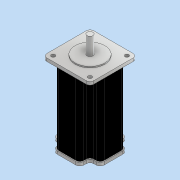
# Autodesk Inventor part: Silnik krokowy SM 60 100-4004AF - 4Nm
Saved by Autodesk Inventor 2018 (Build 220112000, 112)
## iProperties
Created: 2019-01-23
Part Number: Silnik krokowy SM 60 100-4004AF - 4Nm
Material: Ogólny
Document SubType Name: Modeling
Designer: Dawid
Density: 1 g/cm^3
Appearance: Aluminium — ciemne
Author: Dawid
Autodesk Inventor part; units mm, degrees
ref_plane "YZ Plane" through (0, 0, 0) normal (1, 0, 0) x (0, 1, 0)
ref_plane "XZ Plane" through (0, 0, 0) normal (0, 1, 0) x (-1, 0, 0)
ref_plane "XY Plane" through (0, 0, 0) normal (0, 0, 1) x (1, 0, 0)
sketch "Szkic1" plane through (0, 0, 0) normal (0, 0, 1) x (1, 0, 0)
  line L0 (-30, -30) -> (30, -30)
  line L1 (30, -30) -> (30, 30)
  line L2 (30, 30) -> (-30, 30)
  line L3 (-30, 30) -> (-30, -30)
  line L4 (-30, -30) -> (30, 30) construction
  line L5 (30, -30) -> (-30, 30) construction
  point P0 (0, 0)
  dimension "d0" = 60
  dimension "d1" = 60
  constraints: 12 end point, 2 midpoint, 2 parallel, 1 horizontal, 1 perpendicular
  measures "d0" distance of L2.end L1.end
  measures "d1" distance of L1.end L0.end
extrude "Wyciągnięcie proste1" add sketch "Szkic1" along normal blind 100
sketch "Szkic2" plane through (0, 0, 100) normal (0, 0, 1) x (1, 0, 0)
  circle A0 centre (0, 0) radius 19.05
  dimension "d4" = 38.1
  constraints: 1 centre point, 1 coincident
  measures "d4" diameter of A0
extrude "Wyciągnięcie proste2" add sketch "Szkic2" along normal blind 1.6
sketch "Szkic3" plane through (0, 0, 100) normal (0, 0, 1) x (1, 0, 0)
  line L0 (0, 0) -> (0, 23.57)
  line L1 (30, -30) -> (30, 30) projected
  line L2 (-30, 30) -> (-30, -30) projected
  line L3 (0, 0) -> (0, -23.57)
  line L4 (0, -23.57) -> (23.57, -23.57)
  line L5 (0, -23.57) -> (-23.57, -23.57)
  line L6 (0, 23.57) -> (-23.57, 23.57)
  line L7 (0, 23.57) -> (23.57, 23.57)
  circle A0 centre (23.57, 23.57) radius 2.5
  circle A1 centre (-23.57, 23.57) radius 2.5
  circle A2 centre (-23.57, -23.57) radius 2.5
  circle A3 centre (23.57, -23.57) radius 2.5
  dimension "d13" = 47.14
  dimension "d14" = 47.14
  dimension "d15" = 47.14
  dimension "d16" = 5
  dimension "d17" = 5
  dimension "d18" = 5
  dimension "d19" = 5
  constraints: 12 end point, 4 centre point, 4 coincident, 4 horizontal, 1 point on line, 1 vertical
  measures "d13" distance of L7.end L6.end
  measures "d14" distance of L4.end L5.end
  measures "d15" distance of L4.end L7.end
  measures "d16" diameter of A0
  measures "d17" diameter of A1
  measures "d18" diameter of A2
  measures "d19" diameter of A3
extrude "Wyciągnięcie proste3" cut sketch "Szkic3" against normal up to next
sketch "Szkic4" plane through (0, 0, 0) normal (0, 0, -1) x (-1, 0, 0)
  circle A0 centre (23.57, -23.57) radius 2.5 projected
  circle A1 centre (-23.57, 23.57) radius 2.5 projected
  circle A2 centre (23.57, 23.57) radius 2.5 projected
  circle A3 centre (-23.57, -23.57) radius 2.5 projected
  line L0 (30, -30) -> (-30, -30) projected
  line L1 (30, 30) -> (30, -30) projected
  line L2 (-30, 30) -> (30, 30) projected
  line L3 (-30, -30) -> (-30, 30) projected
  line L4 (-30, -30) -> (-30, 30) projected
  line L5 (-17, -17) -> (-17, -30)
  line L6 (17, -17) -> (17, -30)
  line L7 (30, 30) -> (30, -30) projected
  line L8 (-17, -17) -> (-30, -17)
  line L9 (17, 17) -> (30, 17)
  line L10 (-17, 17) -> (-17, 30)
  line L11 (-17, 17) -> (-30, 17)
  line L12 (17, 17) -> (17, 30)
  line L13 (17, -17) -> (30, -17)
  point P0 (0, 0)
  constraints: 16 end point, 8 point on line, 2 parallel, 2 perpendicular
extrude "Wyciągnięcie proste4" cut sketch "Szkic4" against normal blind 96 contours L0 L6 L13 L1 | L0 L3 L8 L5 | L9 L12 L2 L1 | L3 L2 L10 L11
sketch "Szkic5" plane through (0, 0, 101.6) normal (0, 0, 1) x (1, 0, 0)
  circle A0 centre (0, 0) radius 3.75
  dimension "d25" = 7.5
  constraints: 1 centre point, 1 coincident
  measures "d25" diameter of A0
extrude "Wyciągnięcie proste5" add sketch "Szkic5" along normal blind 22.5
sketch "Szkic6" plane through (-30, 30, 100) normal (0, 1, 0) x (1, 0, 0)
  line L0 (13, 100) -> (13, 4) projected
  line L1 (13, 4) -> (0, 4) projected
  line L2 (0, 4) -> (0, 0) projected
  line L3 (60, 0) -> (0, 0) projected
  line L4 (60, 4) -> (60, 0) projected
  line L5 (60, 4) -> (47, 4) projected
  line L6 (47, 4) -> (47, 100) projected
  line L7 (47, 100) -> (13, 100) projected
  line L8 (13, 4) -> (47, 4)
  line L9 (13, 100) -> (13, 4) projected
  line L10 (13, 100) -> (13, 96)
  line L11 (13, 96) -> (47, 96)
  point P0 (30, 100)
  dimension "d28" = 4
  constraints: 6 end point, 2 point on line, 1 horizontal, 1 perpendicular
  measures "d28" distance of L0.start L10.end
extrude "Wyciągnięcie proste6" cut sketch "Szkic6" against normal blind 1 contours L11 L6 L8 L0
sketch "Szkic7" plane through (-30, -30, 100) normal (-1, 0, 0) x (0, 0, 1)
  line L0 (-4, 47) -> (-100, 47) projected
  line L1 (-100, 47) -> (-100, 13) projected
  line L2 (-100, 13) -> (-4, 13) projected
  line L3 (-4, 13) -> (-4, 0) projected
  line L4 (-4, 0) -> (0, 0) projected
  line L5 (0, 60) -> (0, 0) projected
  line L6 (-4, 60) -> (0, 60) projected
  line L7 (-4, 60) -> (-4, 47) projected
  line L8 (-100, 47) -> (-4, 47) projected
  line L9 (-100, 13) -> (-4, 13) projected
  line L10 (-4, 47) -> (-4, 13)
  line L11 (-100, 47) -> (-100, 13) projected
  line L12 (-96, 13) -> (-96, 47)
  point P0 (-100, 30)
  constraints: 4 end point, 2 point on line, 1 perpendicular, 1 vertical
sketch "Szkic8" plane through (-30, -30, 100) normal (0, -1, 0) x (1, 0, 0)
  line L0 (13, -4) -> (13, -100) projected
  line L1 (13, -100) -> (47, -100) projected
  line L2 (47, -100) -> (47, -4) projected
  line L3 (47, -4) -> (60, -4) projected
  line L4 (60, -4) -> (60, 0) projected
  line L5 (0, 0) -> (60, 0) projected
  line L6 (0, -4) -> (0, 0) projected
  line L7 (0, -4) -> (13, -4) projected
  line L8 (47, -4) -> (13, -4) projected
  line L9 (13, -4) -> (47, -4)
  line L10 (47, -100) -> (47, -96)
  line L11 (47, -100) -> (47, -4) projected
  line L12 (47, -96) -> (13, -96)
  point P0 (30, -100)
  dimension "d34" = 4
  constraints: 6 end point, 2 point on line, 1 horizontal, 1 perpendicular
  measures "d34" distance of L1.end L10.end
sketch "Szkic9" plane through (30, -30, 100) normal (1, 0, 0) x (0, 0, -1)
  line L0 (4, 13) -> (100, 13) projected
  line L1 (100, 13) -> (100, 47) projected
  line L2 (100, 47) -> (4, 47) projected
  line L3 (4, 47) -> (4, 60) projected
  line L4 (4, 60) -> (0, 60) projected
  line L5 (0, 0) -> (0, 60) projected
  line L6 (4, 0) -> (0, 0) projected
  line L7 (4, 0) -> (4, 13) projected
  line L8 (4, 47) -> (4, 13) projected
  line L9 (4, 13) -> (4, 47)
  line L10 (100, 47) -> (100, 60) projected
  line L11 (100, 47) -> (96, 47)
  line L12 (100, 47) -> (4, 47) projected
  line L13 (96, 47) -> (96, 13)
  line L14 (100, 13) -> (4, 13) projected
  point P0 (100, 30)
  dimension "d37" = 4
  constraints: 6 end point, 2 point on line, 1 perpendicular, 1 vertical
  measures "d37" distance of L1.end L11.end
extrude "Wyciągnięcie proste10" cut sketch "Szkic8" against normal blind 1 contours L8 L2 L12 L0
extrude "Wyciągnięcie proste11" cut sketch "Szkic7" against normal blind 1 contours L10 L2 L12 L0
extrude "Wyciągnięcie proste12" cut sketch "Szkic9" against normal blind 1 contours L8 L2 L13 L0
sketch "Szkic10" plane through (-30, 17, 0) normal (0, 1, 0) x (1, 0, 0)
  line L0 (1, -4) -> (1, -96)
  line L1 (1, -96) -> (13, -96)
  line L2 (13, -4) -> (13, -96)
  line L3 (1, -4) -> (1, -96)
  line L4 (1, -4) -> (13, -4)
  point P0 (30, 0)
  constraints: 10 end point
extrude "Wyciągnięcie proste13" cut sketch "Szkic10" against normal blind 1
sketch "Szkic11" plane through (-17, 17, 0) normal (-1, 0, 0) x (0, 0, 1)
  line L0 (4, 0) -> (4, -1)
  line L1 (4, -1) -> (96, -1)
  line L2 (96, -1) -> (96, 12)
  line L3 (96, 12) -> (4, 12)
  line L4 (96, 12) -> (4, 12)
  line L5 (4, 12) -> (4, 0)
  point P0 (0, -17)
  constraints: 12 end point
extrude "Wyciągnięcie proste14" cut sketch "Szkic11" against normal blind 1
sketch "Szkic12" plane through (17, 17, 0) normal (0, 1, 0) x (1, 0, 0)
  line L0 (12, -96) -> (12, -4)
  line L1 (0, -4) -> (0, -96)
  line L2 (0, -96) -> (12, -96)
  line L3 (12, -4) -> (0, -4)
  point P0 (-17, 0)
  constraints: 8 end point
extrude "Wyciągnięcie proste15" cut sketch "Szkic12" against normal blind 1
sketch "Szkic13" plane through (17, 17, 0) normal (1, 0, 0) x (0, 0, -1)
  line L0 (-4, 12) -> (-96, 12)
  line L1 (-96, 12) -> (-96, -1)
  line L2 (-96, -1) -> (-4, -1)
  line L3 (-4, 0) -> (-4, -1)
  line L4 (-4, -1) -> (-4, 12)
  line L5 (-4, 0) -> (-4, 12)
  point P0 (0, -17)
  constraints: 12 end point
extrude "Wyciągnięcie proste16" cut sketch "Szkic13" against normal blind 1
sketch "Szkic14" plane through (17, -17, 0) normal (0, -1, 0) x (1, 0, 0)
  line L0 (12, 4) -> (12, 96)
  line L1 (12, 96) -> (0, 96)
  line L2 (0, 4) -> (0, 96)
  line L3 (0, 4) -> (12, 4)
  line L4 (-1, 4) -> (-1, 96)
  point P0 (-17, 0)
  constraints: 10 end point
extrude "Wyciągnięcie proste17" cut sketch "Szkic14" against normal blind 1
sketch "Szkic15" plane through (17, -30, 0) normal (1, 0, 0) x (0, 0, -1)
  line L0 (-96, 1) -> (-4, 1)
  line L1 (-4, 13) -> (-4, 14)
  line L2 (-4, 14) -> (-96, 14)
  line L3 (-96, 14) -> (-96, 1)
  line L4 (-4, 1) -> (-96, 1)
  line L5 (-4, 1) -> (-4, 13)
  point P0 (0, 30)
  constraints: 12 end point
extrude "Wyciągnięcie proste18" cut sketch "Szkic15" against normal blind 1
sketch "Szkic16" plane through (-30, -17, 0) normal (0, -1, 0) x (1, 0, 0)
  line L0 (1, 96) -> (1, 4)
  line L1 (13, 4) -> (13, 96)
  line L2 (13, 96) -> (1, 96)
  line L3 (1, 4) -> (14, 4)
  line L4 (13, 4) -> (1, 4)
  point P0 (30, 0)
  constraints: 10 end point, 1 point on line
extrude "Wyciągnięcie proste19" cut sketch "Szkic16" against normal blind 1
sketch "Szkic17" plane through (-17, -30, 0) normal (-1, 0, 0) x (0, 0, 1)
  line L0 (4, 1) -> (96, 1)
  line L1 (96, 1) -> (96, 14)
  line L2 (96, 14) -> (4, 14)
  line L3 (4, 13) -> (4, 14)
  line L4 (4, 14) -> (4, 1)
  line L5 (4, 13) -> (4, 1)
  point P0 (0, 30)
  constraints: 12 end point
extrude "Wyciągnięcie proste20" cut sketch "Szkic17" against normal blind 1
fillet "Zaokrąglenie1" radius 5 28 edges at (-30, 30, 98) (30, 30, 98) (30, -30, 98) (-30, -30, 98) (-16, -16, 50) (-29, -16, 50) (-16, -29, 50) (16, -29, 50) (16, -16, 50) (29, -16, 50) (29, 16, 50) (16, 16, 50) (16, 29, 50) (-16, 29, 50) (-16, 16, 50) (-29, 16, 50) (-30, 17, 2) (-17, 17, 2) (-17, 30, 2) (17, 30, 2) (17, 17, 2) (30, 17, 2) (30, -17, 2) (17, -17, 2) (17, -30, 2) (-17, -30, 2) (-17, -17, 2) (-30, -17, 2)
